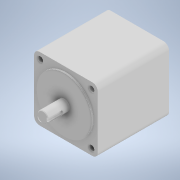
# Autodesk Inventor part: Motor 1KW
Saved by Autodesk Inventor 2022 (Build 260153000, 153)
## iProperties
Created: 2021-09-10
Part Number: Motor 1KW
Material: Generic
Document SubType Name: Modeling
Designer: ARMU
Density: 1 g/cm^3
Appearance: Default
Author: ARMU
Autodesk Inventor part; units mm, degrees
ref_plane "YZ Plane" through (0, 0, 0) normal (1, 0, 0) x (0, 1, 0)
ref_plane "XZ Plane" through (0, 0, 0) normal (0, 1, 0) x (-1, 0, 0)
ref_plane "XY Plane" through (0, 0, 0) normal (0, 0, 1) x (1, 0, 0)
sketch "Sketch1" plane through (0, 0, 0) normal (0, 0, 1) x (1, 0, 0)
  line L0 (-55, 55) -> (55, 55)
  line L1 (55, 55) -> (55, -55)
  line L2 (55, -55) -> (-55, -55)
  line L3 (-55, -55) -> (-55, 55)
  line L4 (-55, 55) -> (55, -55) construction
  line L5 (55, 55) -> (-55, -55) construction
  point P0 (0, 0)
  dimension "d0" = 110
  dimension "d1" = 110
  constraints: 12 end point, 2 midpoint, 2 parallel, 1 horizontal, 1 perpendicular
  measures "d0" distance of L1.end L2.end
  measures "d1" distance of L0.end L1.end
extrude "Extrusion1" add sketch "Sketch1" along normal blind 123
sketch "Sketch2" plane through (0, 0, 123) normal (0, 0, 1) x (1, 0, 0)
  circle A0 centre (0, 0) radius 62.5 construction
  line L0 (55, -55) -> (55, 55) construction
  line L1 (0, 0) -> (55, 55) construction
  line L2 (0, 0) -> (77.7817, 0) construction
  circle A1 centre (44.1942, 44.1942) radius 4.75
  circle A2 centre (-44.1942, 44.1942) radius 4.75
  circle A3 centre (-44.1942, -44.1942) radius 4.75
  circle A4 centre (44.1942, -44.1942) radius 4.75
  dimension "d4" = 125
  dimension "d5" = 45
  dimension "d6" = 9.5
  dimension "d9" = 360
  constraints: 4 centre point, 4 end point, 1 coincident, 1 equal length, 1 horizontal, 1 point on line, 12 other
  measures "d5" angle of L2 L1
  measures "d6" diameter of A1
extrude "Extrusion2" cut sketch "Sketch2" against normal blind 123
sketch "Sketch3" plane through (0, 0, 123) normal (0, 0, 1) x (1, 0, 0)
  circle A0 centre (0, 0) radius 47.5
  dimension "d13" = 95
  constraints: 1 centre point, 1 coincident
  measures "d13" diameter of A0
extrude "Extrusion3" add sketch "Sketch3" along normal blind 3
sketch "Sketch4" plane through (0, 0, 126) normal (0, 0, 1) x (1, 0, 0)
  circle A0 centre (0, 0) radius 9.5
  dimension "d16" = 19
  constraints: 1 centre point, 1 coincident
  measures "d16" diameter of A0
extrude "Extrusion4" add sketch "Sketch4" along normal blind 37
fillet "Fillet1" radius 9.5 4 edges at (55, 55, 61.5) (-55, 55, 61.5) (-55, -55, 61.5) (55, -55, 61.5)
chamfer "Chamfer1" distance 1 angle 45 1 edges at (-9.5, 0, 163)
sketch "Sketch5" plane through (0, 0, 163) normal (0, 0, 1) x (1, 0, 0)
  circle A0 centre (0, 0) radius 8.5 construction
  line L0 (-8.5, 0) -> (-8.5, 20.2079) construction
  line L1 (6.9, 3) -> (12.9, 3)
  line L2 (12.9, 3) -> (12.9, -3)
  line L3 (12.9, -3) -> (6.9, -3)
  line L4 (6.9, -3) -> (6.9, 3)
  line L5 (6.9, 3) -> (12.9, -3) construction
  line L6 (12.9, 3) -> (6.9, -3) construction
  line L7 (0, 0) -> (24.5992, 0) construction
  line L8 (0, 0) -> (24.5992, 0) construction
  line L9 (0, 0) -> (-9.5, 0) construction
  circle A1 centre (0, 0) radius 9.5 construction
  point P0 (9.9, 0)
  dimension "d23" = 6
  dimension "d24" = 6
  dimension "d25" = 0
  dimension "d26" = 22.4
  constraints: 20 end point, 3 horizontal, 2 horizontal alignment, 2 parallel, 2 vertical, 1 collinear, 1 midpoint, 1 perpendicular, 1 point on line, 2 other
  measures "d23" distance of L2.end L3.end
  measures "d24" distance of L1.end L2.end
  measures "d25" distance between parallel lines of L7 L8
  measures "d26" distance from line of L2 L9.end
extrude "Extrusion5" cut sketch "Sketch5" against normal blind 25
fillet "Fillet2" radius 3 2 edges at (7.9569, -3, 138) (7.9569, 3, 138)
body "Solid1"
